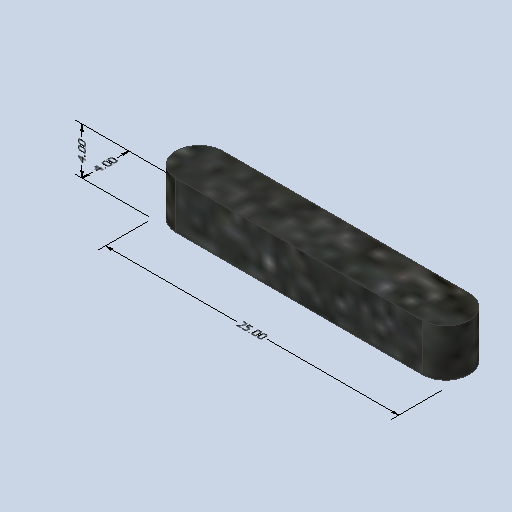
# Autodesk Inventor part: KKES04-025
Saved by Autodesk Inventor 2023 (Build 270158000, 158)
## iProperties
Category: PARTsolutions
Company: TOHATSU
Created: 2023-07-21
Part Number: KKES04-025
Material: Steel
Catalog Web Link: www.cadenas.de
Description: KKED、KKES、KKEG-parallel key
Vendor: TOHATSU
Document SubType Name: Modeling
Designer: psAdmin
Manufacturer: TOHATSU
Mass: 3.03218 g
Surface Area: 4.11398 cm^2
Volume: 0.386265 cm^3
Density: 7.85 g/cm^3
Appearance: Plate
PSOL_IDENT_0: {$CADENAS_DATA/23d-libs/tohatsu/machinery-components/locating-fixed-components/machine_keys/kke.prj}
PSOL_IDENT_1: ,182 {VTYP=3D},{NB=KKES04-025},{LINA=KKES04-025},{NN=KKED、KKES、KKEG},{DATE=19.07.2023 02:54:23},{GEO
PSOL_IDENT_2: MDATE=29.05.2023 08:31:00},{VERSION=},{LINEID=10},{WBVAR=TYPE,MA,B,L},{WBNUMERIC=B,L}  {NB=KKES04-02
PSOL_IDENT_3: 5},{LINA=KKES04-025},{KT=DUMMY},{PN=KKES04-025},{TYPE=KKES},{MA=S45C},{CO=0.73,0.75,0.79,0.00},{ROHS=
PSOL_IDENT_4: YES},{QU=7850},{B=4},{DIMB=04},{L=25},{DIMLL=025},{DIML=8,10,12,15,16,18,20,25,30,35,40,45,50},{H=4}
PSOL_IDENT_5: ,{C=0.16},{WED=網站},{URL=https://www.tohatsu.com.tw}
NB: KKES04-025
NN: KKED、KKES、KKEG
NT: parallel key
NBSYN: $PN.
LINA: KKES04-025
CATALOG: TOHATSU
PN: KKES04-025
TYPE: KKES
MA: S45C
ROHS: YES
B: 4
L: 25
H: 4
WED: 網站
SUPPLIER: TOHATSU
ARTICLENO: KKES04-025
BOMINFO: KKES04-025
CREATOR: CADENAS GmbH
Title: KKES04-025
Author: Cadenas PARTsolutions
Comments: parallel key
Autodesk Inventor part; units mm, degrees
ref_plane "YZ Plane" through (0, 0, 0) normal (1, 0, 0) x (0, 1, 0)
ref_plane "XZ Plane" through (0, 0, 0) normal (0, 1, 0) x (-1, 0, 0)
ref_plane "XY Plane" through (0, 0, 0) normal (0, 0, 1) x (1, 0, 0)
sketch "__1" plane through (0, 0, 0) normal (0, 1, 0) x (-1, 0, 0)
  line L0 (0, -4) -> (0, 0)
  line L1 (0, 0) -> (-25, 0)
  line L2 (-25, 0) -> (-25, -4)
  line L3 (-25, -4) -> (0, -4)
  constraints: 8 end point
extrude "Extrusion1" add sketch "__1" along normal blind 4
fillet "Fillet1" radius 2 4 edges at (0, 2, -4) (25, 2, -4) (25, 2, 0) (0, 2, 0)
body "Solid1"
